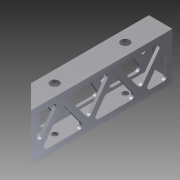
# Autodesk Inventor part: left fram piece 3
Saved by Autodesk Inventor 2012 (Build 160160000, 160)
## iProperties
Created: 2013-01-04
Part Number: left fram piece 3
Material: Default
Document SubType Name: Modeling
Designer: Bryce
Density: 1 g/cm^3
Author: Bryce
Autodesk Inventor part; units mm, degrees
ref_plane "YZ Plane" through (0, 0, 0) normal (1, 0, 0) x (0, 1, 0)
ref_plane "XZ Plane" through (0, 0, 0) normal (0, 1, 0) x (-1, 0, 0)
ref_plane "XY Plane" through (0, 0, 0) normal (0, 0, 1) x (1, 0, 0)
sketch "Sketch1" plane through (0, 0, 0) normal (0, 0, 1) x (1, 0, 0)
  line L0 (0, 0) -> (25.4, 0)
  line L1 (25.4, 0) -> (25.4, 50.8)
  line L2 (25.4, 50.8) -> (0, 50.8)
  line L3 (0, 50.8) -> (0, 0)
  line L4 (3.175, 3.175) -> (22.225, 3.175)
  line L5 (22.225, 3.175) -> (22.225, 47.625)
  line L6 (22.225, 47.625) -> (3.175, 47.625)
  line L7 (3.175, 47.625) -> (3.175, 3.175)
  dimension "d0" = 50.8
  dimension "d1" = 25.4
  dimension "d2" = 3.175
  dimension "d3" = 3.175
  dimension "d4" = 3.175
  dimension "d5" = 3.175
  constraints: 16 end point, 4 parallel, 2 horizontal, 2 perpendicular
  measures "d0" distance of L0.end L1.end
  measures "d1" distance of L1.end L2.end
  measures "d2" distance between parallel lines of L6 L2
  measures "d3" distance between parallel lines of L1 L5
  measures "d4" distance between parallel lines of L0 L4
  measures "d5" distance between parallel lines of L3 L7
extrude "Extrusion1" add sketch "Sketch1" along normal blind 152.4
sketch "Sketch2" plane through (0, 0, 0) normal (0, -1, 0) x (1, 0, 0)
  line L0 (25.4, 152.4) -> (0, 152.4) projected
  line L1 (0, 0) -> (0, 152.4) projected
  line L2 (25.4, 0) -> (25.4, 152.4) projected
  line L3 (0, 152.4) -> (25.4, 127)
  circle A0 centre (12.7, 114.3) radius 3.175
  circle A1 centre (12.7, 38.1) radius 3.175
  dimension "d8" = 45
  dimension "d9" = 6.35
  dimension "d10" = 12.7
  dimension "d11" = 38.1
  dimension "d12" = 76.2
  constraints: 2 centre point, 2 end point, 1 equal radius, 1 point on line, 1 vertical alignment
  measures "d8" angle of L3 L0
  measures "d9" diameter of A0
  measures "d10" distance from line of L1 A0.centre
  measures "d11" distance from line of L0 A0.centre
  measures "d12" distance of A1.centre A0.centre
extrude "Extrusion2" cut sketch "Sketch2" against normal blind 3.175 contours A0 | A1
extrude "Extrusion3" cut sketch "Sketch2" against normal through all contours L2 L3 L0
mirror "Mirror1" about plane through (25.4, 50.8, 0) normal (1, 0, 0) remove original yes
sketch "Sketch3" plane through (25.4, 50.8, 0) normal (0, 1, 0) x (1, 0, 0)
  circle A0 centre (12.7, -114.3) radius 4.7625
  circle A1 centre (12.7, -38.1) radius 4.7625
  circle A2 centre (12.7, -38.1) radius 3.175 projected
  circle A3 centre (12.7, -114.3) radius 3.175 projected
  point P0 (-25.4, 0)
  dimension "d17" = 9.525
  constraints: 2 centre point, 2 coincident, 1 equal radius
  measures "d17" diameter of A0
extrude "Extrusion4" cut sketch "Sketch3" against normal blind 25.4 contours A0 | A1 | A2 | A3
sketch "Sketch4" plane through (25.4, 0, 0) normal (-1, 0, 0) x (0, 0, 1)
  line L0 (127, 50.8) -> (127, 0) projected
  line L1 (0, 50.8) -> (127, 50.8) projected
  line L2 (0, 0) -> (0, 50.8) projected
  line L3 (0, 0) -> (127, 0) projected
  line L4 (74.93, 38.2789) -> (55.7727, 6.35)
  line L5 (52.07, 6.35) -> (74.93, 44.45) construction
  line L6 (6.35, 6.35) -> (120.65, 6.35)
  line L7 (120.65, 44.45) -> (6.35, 44.45)
  line L8 (71.2273, 44.45) -> (52.07, 12.5211)
  line L9 (74.93, 38.2789) -> (94.0873, 6.35)
  line L10 (74.93, 44.45) -> (97.79, 6.35) construction
  line L11 (78.6327, 44.45) -> (97.79, 12.5211)
  line L12 (97.79, 12.5211) -> (116.9473, 44.45)
  line L13 (97.79, 6.35) -> (120.65, 44.45) construction
  line L14 (101.4927, 6.35) -> (120.65, 38.2789)
  line L15 (120.65, 6.35) -> (120.65, 44.45)
  line L16 (6.35, 44.45) -> (6.35, 6.35)
  line L17 (6.35, 6.35) -> (29.21, 44.45) construction
  line L18 (32.9127, 44.45) -> (52.07, 12.5211)
  line L19 (29.21, 44.45) -> (52.07, 6.35) construction
  line L20 (48.3673, 6.35) -> (29.21, 38.2789)
  line L21 (10.0527, 6.35) -> (29.21, 38.2789)
  line L22 (6.35, 12.5211) -> (25.5073, 44.45)
  dimension "d20" = 30.964
  dimension "d21" = 61.928
  dimension "d22" = 61.928
  dimension "d23" = 61.928
  dimension "d24" = 61.928
  dimension "d25" = 3.175
  dimension "d26" = 3.175
  dimension "d27" = 3.175
  dimension "d28" = 3.175
  dimension "d29" = 3.175
  dimension "d30" = 3.175
  dimension "d31" = 3.175
  dimension "d32" = 3.175
  dimension "d33" = 3.175
  dimension "d34" = 3.175
  dimension "d35" = 6.35
  dimension "d36" = 6.35
  dimension "d37" = 6.35
  dimension "d38" = 6.35
  constraints: 34 end point, 8 parallel, 2 point on line, 1 vertical, 20 other
  measures "d20" angle of L17 L16
  measures "d21" angle of L19 L17
  measures "d22" angle of L5 L19
  measures "d23" angle of L10 L5
  measures "d24" angle of L13 L10
  measures "d25" distance between parallel lines of L17 L22
  measures "d26" distance between parallel lines of L17 L21
  measures "d27" distance between parallel lines of L19 L20
  measures "d28" distance between parallel lines of L18 L19
  measures "d29" distance between parallel lines of L5 L8
  measures "d30" distance between parallel lines of L5 L4
  measures "d31" distance between parallel lines of L10 L9
  measures "d32" distance between parallel lines of L10 L11
  measures "d33" distance between parallel lines of L13 L12
  measures "d34" distance between parallel lines of L14 L13
  measures "d35" distance between parallel lines of L0 L15
  measures "d38" distance between parallel lines of L2 L16
extrude "Extrusion5" cut sketch "Sketch4" against normal blind 3.175 contours L9 L6 L4 | L6 L21 L20 | L14 L15 L6 | L16 L7 L22 | L12 L11 L7 | L7 L8 L18
sketch "Sketch5" plane through (50.8, 0, 0) normal (1, 0, 0) x (0, 0, -1)
  line L0 (-152.4, 0) -> (-152.4, 50.8) projected
  line L1 (0, 0) -> (-152.4, 0) projected
  line L2 (0, 50.8) -> (0, 0) projected
  line L3 (0, 50.8) -> (-152.4, 50.8) projected
  line L4 (-66.1672, 44.45) -> (-90.17, 11.7189)
  line L5 (-90.17, 6.35) -> (-62.23, 44.45) construction
  line L6 (-146.05, 6.35) -> (-6.35, 6.35)
  line L7 (-6.35, 44.45) -> (-146.05, 44.45)
  line L8 (-62.23, 39.0811) -> (-86.2328, 6.35)
  line L9 (-62.23, 44.45) -> (-34.29, 6.35) construction
  line L10 (-58.2928, 44.45) -> (-34.29, 11.7189)
  line L11 (-114.1728, 44.45) -> (-90.17, 11.7189)
  line L12 (-118.11, 44.45) -> (-90.17, 6.35) construction
  line L13 (-94.1072, 6.35) -> (-118.11, 39.0811)
  line L14 (-62.23, 39.0811) -> (-38.2272, 6.35)
  line L15 (-142.1128, 6.35) -> (-118.11, 39.0811)
  line L16 (-146.05, 44.45) -> (-146.05, 6.35)
  line L17 (-146.05, 6.35) -> (-118.11, 44.45) construction
  line L18 (-146.05, 11.7189) -> (-122.0472, 44.45)
  line L19 (-34.29, 11.7189) -> (-10.2872, 44.45)
  line L20 (-30.3528, 6.35) -> (-6.35, 39.0811)
  line L21 (-6.35, 6.35) -> (-6.35, 44.45)
  line L22 (-34.29, 6.35) -> (-6.35, 44.45) construction
  dimension "d41" = 36.254
  dimension "d42" = 72.508
  dimension "d43" = 72.508
  dimension "d44" = 72.508
  dimension "d45" = 72.508
  dimension "d46" = 3.175
  dimension "d47" = 3.175
  dimension "d48" = 3.175
  dimension "d49" = 3.175
  dimension "d50" = 3.175
  dimension "d51" = 3.175
  dimension "d52" = 3.175
  dimension "d53" = 3.175
  dimension "d54" = 3.175
  dimension "d55" = 3.175
  dimension "d56" = 6.35
  dimension "d57" = 6.35
  dimension "d58" = 6.35
  dimension "d59" = 6.35
  constraints: 34 end point, 8 parallel, 2 point on line, 1 vertical, 20 other
  measures "d41" angle of L17 L16
  measures "d42" angle of L12 L17
  measures "d43" angle of L5 L12
  measures "d44" angle of L9 L5
  measures "d45" angle of L22 L9
  measures "d46" distance between parallel lines of L17 L18
  measures "d47" distance between parallel lines of L17 L15
  measures "d48" distance between parallel lines of L12 L13
  measures "d49" distance between parallel lines of L11 L12
  measures "d50" distance between parallel lines of L5 L4
  measures "d51" distance between parallel lines of L5 L8
  measures "d52" distance between parallel lines of L9 L14
  measures "d53" distance between parallel lines of L9 L10
  measures "d54" distance between parallel lines of L22 L19
  measures "d55" distance between parallel lines of L20 L22
  measures "d56" distance between parallel lines of L0 L16
  measures "d58" distance between parallel lines of L2 L21
extrude "Extrusion6" cut sketch "Sketch5" against normal blind 3.175 contours L4 L11 L7 | L7 L19 L10 | L18 L16 L7 | L21 L6 L20 | L15 L13 L6 | L6 L8 L14
fillet "Fillet1" radius 3.175 36 edges at (49.2125, 11.7189, 146.05) (49.2125, 44.45, 146.05) (49.2125, 44.45, 122.0472) (49.2125, 39.0811, 118.11) (49.2125, 6.35, 142.1128) (49.2125, 6.35, 94.1072) (49.2125, 11.7189, 90.17) (49.2125, 44.45, 114.1728) (49.2125, 44.45, 66.1672) (49.2125, 39.0811, 62.23) (49.2125, 6.35, 38.2272) (49.2125, 6.35, 86.2328) (49.2125, 11.7189, 34.29) (49.2125, 44.45, 58.2928) (49.2125, 44.45, 10.2872) (49.2125, 39.0811, 6.35) (49.2125, 6.35, 30.3528) (49.2125, 6.35, 6.35) (26.9875, 12.5211, 6.35) (26.9875, 6.35, 10.0527) (26.9875, 38.2789, 29.21) (26.9875, 44.45, 25.5073) (26.9875, 6.35, 48.3673) (26.9875, 44.45, 6.35) (26.9875, 44.45, 32.9127) (26.9875, 12.5211, 52.07) (26.9875, 44.45, 71.2273) (26.9875, 6.35, 94.0873) (26.9875, 6.35, 55.7727) (26.9875, 38.2789, 74.93) (26.9875, 12.5211, 97.79) (26.9875, 44.45, 78.6327) (26.9875, 6.35, 101.4927) (26.9875, 44.45, 116.9473) (26.9875, 6.35, 120.65) (26.9875, 38.2789, 120.65)
equation "\"d3\" = d2"
equation "\"d4\" = d3"
equation "\"d5\" = d4"
equation "\"d21\" = 2 * d20"
equation "\"d22\" = d21"
equation "\"d23\" = d22"
equation "\"d24\" = d23"
equation "\"d26\" = d25"
equation "\"d27\" = d26"
equation "\"d28\" = d27"
equation "\"d29\" = d28"
equation "\"d30\" = d29"
equation "\"d31\" = d30"
equation "\"d32\" = d30"
equation "\"d33\" = d32"
equation "\"d34\" = d33"
equation "\"d42\" = 2 * d41"
equation "\"d43\" = d42"
equation "\"d44\" = d43"
equation "\"d45\" = d44"
equation "\"d47\" = d46"
equation "\"d48\" = d47"
equation "\"d49\" = d48"
equation "\"d50\" = d49"
equation "\"d51\" = d50"
equation "\"d52\" = d51"
equation "\"d53\" = d51"
equation "\"d54\" = d53"
equation "\"d55\" = d54"
body "Solid1"
